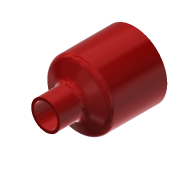
# Autodesk Inventor part: 01_Connector_T
Saved by Autodesk Inventor 2019.4 (Build 234330000, 330)
## iProperties
Created: 2021-06-01
Part Number: 01_Connector_T
Material: Generic
Document SubType Name: Modeling
Designer: diederichbenedict
Density: 1 g/cm^3
Appearance: Smooth - Red
Author: diederichbenedict
Autodesk Inventor part; units mm, degrees
ref_plane "YZ Plane" through (0, 0, 0) normal (1, 0, 0) x (0, 1, 0)
ref_plane "XZ Plane" through (0, 0, 0) normal (0, 1, 0) x (-1, 0, 0)
ref_plane "XY Plane" through (0, 0, 0) normal (0, 0, 1) x (1, 0, 0)
sketch "Sketch1" plane through (0, 0, 0) normal (1, 0, 0) x (0, 1, 0)
  line L0 (9.9, 0) -> (6.6104, -37.6)
  line L1 (11, 0) -> (11, -20)
  line L2 (-11, 0) -> (11, 0) projected
  line L3 (9.115, -8.5875) -> (0, -8.5875)
  line L4 (0, -8.5875) -> (0, 9)
  line L5 (0, 9) -> (4, 9)
  line L6 (4, 9) -> (11, 0) construction
  line L7 (4, 9) -> (9.115, 7)
  line L8 (9.115, 7) -> (9.115, 2)
  line L9 (9.115, 2) -> (9.115, 0)
  line L10 (4, 9) -> (0, 9)
  line L11 (0, 9) -> (0, 16)
  line L12 (0, 16) -> (4, 16)
  line L13 (4, 16) -> (4, 9)
  line L14 (9.115, -8.5875) -> (9.115, 0)
  point P0 (0, 0)
  dimension "d12" = 4
  dimension "d13" = 0
  dimension "d15" = 9.115
  dimension "d16" = 0
  dimension "d17" = 2
  dimension "d19" = 5
  dimension "d20" = 7
  constraints: 28 end point, 4 parallel, 3 perpendicular, 2 horizontal, 2 point on line, 1 vertical, 5 other
  measures "d12" distance between parallel lines of L13 L11
  measures "d13" distance from line of point (0, 0) L4
  measures "d15" distance of L3.end L3.start
  measures "d16" angle of L4 L14
  measures "d17" distance from line of L7.end L5
  measures "d19" distance of L8.end L7.end
  measures "d20" distance between parallel lines of L5 L12
revolve "Revolution1" add sketch "Sketch1" angle 360 about axis through (0, 0, -8.5875) along (0, 0, 1)
sketch "Sketch4" plane through (0, 0, 16) normal (0, 0, 1) x (1, 0, 0)
  circle A0 centre (0, 0) radius 1.4796 projected
  circle A1 centre (0, 0) radius 4 projected
  circle A2 centre (0, 0) radius 3.25
  point P0 (0, 0)
  dimension "d21" = 6.5
  constraints: 1 centre point, 1 coincident
  measures "d21" diameter of A2
extrude "Extrusion2" cut sketch "Sketch4" against normal through all contours A0 | A2
fillet "Fillet2" radius 2 2 edges at (0, -4, 9) (0, -9.115, 7)
body "Solid1"
